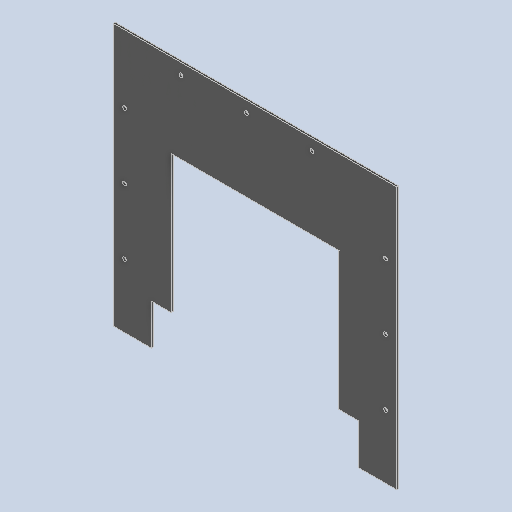
# Autodesk Inventor part: HCMUTE-CDT23-KXL_A04
Saved by Autodesk Inventor 2023 (Build 270158000, 158)
## iProperties
Created: 2023-11-20
Part Number: HCMUTE-CDT23-KXL_A04
Material: PMMA Plastic
Document SubType Name: Modeling
Designer: havie
Density: 1.188 g/cm^3
Appearance: Dark Gray
Author: havie
Autodesk Inventor part; units mm, degrees
ref_plane "YZ Plane" through (0, 0, 0) normal (1, 0, 0) x (0, 1, 0)
ref_plane "XZ Plane" through (0, 0, 0) normal (0, 1, 0) x (-1, 0, 0)
ref_plane "XY Plane" through (0, 0, 0) normal (0, 0, 1) x (1, 0, 0)
sketch "Sketch1" plane through (0, 0, 0) normal (1, 0, 0) x (0, 1, 0)
  line L0 (-216, 200) -> (216, 200)
  line L1 (216, 200) -> (216, -200)
  line L2 (216, -200) -> (-216, -200)
  line L3 (-216, -200) -> (-216, 200)
  line L4 (-216, 200) -> (216, -200) construction
  line L5 (216, 200) -> (-216, -200) construction
  point P0 (0, 0)
  dimension "d0" = 432
  dimension "d1" = 400
  constraints: 12 end point, 2 midpoint, 2 parallel, 1 horizontal, 1 perpendicular
  measures "d0" distance of L1.end L2.end
  measures "d1" distance of L0.end L1.end
extrude "Extrusion1" add sketch "Sketch1" along normal mid plane 3
sketch "Sketch2" plane through (1.5, 0, 0) normal (1, 0, 0) x (0, 0, -1)
  line L0 (200, -216) -> (200, 216) projected
  line L1 (200, -158) -> (138, -158)
  line L2 (138, -158) -> (138, -128)
  line L3 (138, -128) -> (-72, -128)
  line L4 (-72, -128) -> (-72, 128)
  line L5 (-72, 128) -> (138, 128)
  line L6 (138, 128) -> (138, 158)
  line L7 (138, 158) -> (200, 158)
  line L8 (-200, -216) -> (200, -216) projected
  line L9 (200, 216) -> (-200, 216) projected
  point P0 (0, 0)
  dimension "d4" = 58
  dimension "d5" = 58
  dimension "d6" = 62
  dimension "d7" = 30
  dimension "d8" = 210
  constraints: 14 end point, 6 perpendicular, 2 equal length, 2 point on line, 1 horizontal
  measures "d4" distance between parallel lines of L8 L1
  measures "d5" distance between parallel lines of L9 L7
  measures "d6" distance of L1.start L1.end
  measures "d7" distance of L1.end L2.end
  measures "d8" distance between parallel lines of L4 L2
extrude "Extrusion2" cut sketch "Sketch2" against normal blind 3
sketch "Sketch3" plane through (1.5, 0, 0) normal (1, 0, 0) x (0, 0, -1)
  circle A0 centre (3, 199) radius 3
  circle A1 centre (103, 199) radius 3
  circle A2 centre (-97, 199) radius 3
  circle A3 centre (-97, -199) radius 3
  circle A4 centre (3, -199) radius 3
  circle A5 centre (103, -199) radius 3
  line L0 (-200, 216) -> (-200, -216) projected
  line L1 (200, 216) -> (-200, 216) projected
  line L2 (-200, -216) -> (200, -216) projected
  point P0 (0, 0)
  dimension "d13" = 103
  dimension "d14" = 17
  dimension "d15" = 6
  dimension "d16" = 100
  dimension "d17" = 100
  dimension "d18" = 17
  dimension "d19" = 100
  constraints: 6 centre point, 5 equal radius, 4 horizontal alignment, 2 vertical alignment
  measures "d13" distance from line of L0 A2.centre
  measures "d14" distance from line of L1 A2.centre
  measures "d15" diameter of A2
  measures "d16" distance of A2.centre A0.centre
  measures "d17" distance of A1.centre A0.centre
  measures "d18" distance from line of L2 A3.centre
  measures "d19" distance of A4.centre A5.centre
extrude "Extrusion3" cut sketch "Sketch3" against normal blind 3
sketch "Sketch4" plane through (1.5, 0, 0) normal (1, 0, 0) x (0, 0, -1)
  circle A0 centre (-183, -113) radius 2.5 projected
  circle A1 centre (-183, -13) radius 2.5 projected
  arc A2 (-183, 79.5) -> (-183, 94.5) centre (-183, 87) ccw projected
  line L0 (-183, 94.5) -> (-194, 94.5) projected
  line L1 (-194, 79.5) -> (-194, 94.5) projected
  line L2 (-183, 79.5) -> (-194, 79.5) projected
  circle A3 centre (-183, 87) radius 2.5 projected
  point P0 (0, 0)
  constraints: 3 coincident
hole "Hole1" at (1.5, -113, 183) at (1.5, -13, 183) at (1.5, 87, 183) direction (-1, 0, 0) diameter 6 depth 14.2 tip angle 118
equation "\"d5\" = d4"
body "Solid1"
